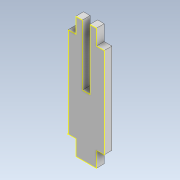
# Autodesk Inventor part: bracket
Saved by Autodesk Inventor 2022 (Build 260153000, 153)
## iProperties
Created: 2023-05-02
Part Number: bracket
Material: 一般
Document SubType Name: Modeling
Designer: JOU
Density: 1 g/cm^3
Appearance: 預設
Author: JOU
Autodesk Inventor part; units mm, degrees
ref_plane "YZ Plane" through (0, 0, 0) normal (1, 0, 0) x (0, 1, 0)
ref_plane "XZ Plane" through (0, 0, 0) normal (0, 1, 0) x (-1, 0, 0)
ref_plane "XY Plane" through (0, 0, 0) normal (0, 0, 1) x (1, 0, 0)
sketch "草圖1" plane through (0, 0, 0) normal (0, 0, 1) x (1, 0, 0)
  line L0 (0, 35) -> (14, 35)
  line L1 (14, 35) -> (14, 0)
  line L2 (14, 0) -> (0, 0)
  line L3 (0, 0) -> (0, 35)
  line L4 (3, 0) -> (11, 0)
  line L5 (11, 0) -> (11, -6)
  line L6 (11, -6) -> (3, -6)
  line L7 (3, -6) -> (3, 0)
  line L8 (3, 35) -> (11, 35)
  line L9 (11, 35) -> (11, 41)
  line L10 (11, 41) -> (3, 41)
  line L11 (3, 41) -> (3, 35)
  point P0 (11, 0)
  dimension "d0" = 14
  dimension "d1" = 6
  dimension "d2" = 8
  dimension "d3" = 3
  dimension "d4" = 35
  dimension "d5" = 6
  constraints: 24 end point, 6 parallel, 3 horizontal, 3 perpendicular, 2 collinear, 2 point on line, 1 coincident
  measures "d0" distance between parallel lines of L3 L1
  measures "d1" distance of L4.end L5.end
  measures "d2" distance between parallel lines of L7 L5
  measures "d3" distance between parallel lines of L3 L7
  measures "d4" distance of L0.end L1.end
  measures "d5" distance of L8.end L9.end
extrude "擠出1" add sketch "草圖1" along normal blind 3
sketch "草圖2" plane through (0, 0, 3) normal (0, 0, 1) x (1, 0, 0)
  line L0 (11, 41) -> (3, 41) projected
  line L1 (5.55, 41) -> (8.45, 41)
  line L2 (8.45, 41) -> (8.45, 17.5)
  line L3 (8.45, 17.5) -> (5.55, 17.5)
  line L4 (5.55, 17.5) -> (5.55, 41)
  line L5 (3, 41) -> (3, 35) projected
  line L6 (3, -6) -> (11, -6) projected
  point P0 (0, 0)
  dimension "d8" = 2.9
  dimension "d9" = 2.55
  dimension "d10" = 23.5
  dimension "d13" = 47
  constraints: 8 end point, 2 parallel, 1 horizontal, 1 perpendicular, 1 point on line
  measures "d8" distance between parallel lines of L4 L2
  measures "d9" distance between parallel lines of L5 L4
  measures "d10" distance of L1.end L2.end
  measures "d13" distance between parallel lines of L6 L0
extrude "擠出2" cut sketch "草圖2" against normal up to surface (3 mm away)
sketch "草圖3" plane through (0, 0, 3) normal (0, 0, 1) x (1, 0, 0)
  line L0 (5.55, 17.5) -> (5.55, 41) projected
  line L1 (5.55, 41) -> (3, 41) projected
  line L2 (3, 41) -> (3, 35) projected
  line L3 (3, 35) -> (0, 35) projected
  line L4 (0, 35) -> (0, 0) projected
  line L5 (0, 0) -> (3, 0) projected
  line L6 (3, 0) -> (3, -6) projected
  line L7 (3, -6) -> (11, -6) projected
  line L8 (11, -6) -> (11, 0) projected
  line L9 (11, 0) -> (14, 0) projected
  line L10 (14, 0) -> (14, 35) projected
  line L11 (14, 35) -> (11, 35) projected
  line L12 (11, 35) -> (11, 41) projected
  line L13 (11, 41) -> (8.45, 41) projected
  line L14 (8.45, 41) -> (8.45, 17.5) projected
  line L15 (8.45, 17.5) -> (5.55, 17.5) projected
equation "\"d10\" = 0.5 * d13"
